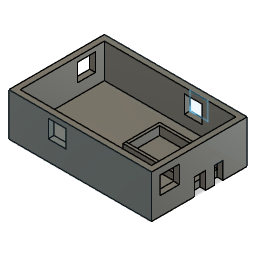
PDT LED Original Bottom Array Case v4 (Autodesk Fusion 360 design; units mm, degrees)
Autodesk Fusion 360 part; units mm, degrees
sketch "Sketch1" plane through (0, 0, 0) normal (0, 1, 0) x (1, 0, 0)
  line L0 (0, 0) -> (250, 0)
  line L1 (250, 0) -> (250, -150)
  line L2 (250, -150) -> (0, -150)
  line L3 (0, -150) -> (0, 0)
  constraint horizontal L0
  constraint vertical L1
  constraint horizontal L2
  constraint vertical L3
  constraint coincident L0.start L3.end
extrude "Extrude1" add sketch "Sketch1" along normal blind 75 makes body 1
move_face "OffsetFaces1" offset 17.253 1 faces at (83.3333, 25, 0) on bodies 1
shell "Shell1" thickness 10 removed faces 1 at (83.3333, 75, 38.498) on bodies 1
sketch "Sketch2" plane through (0, 10, 0) normal (0, 1, 0) x (-1, 0, 0)
  line L0 (-10, 140) -> (-240, 140)
  line L1 (-240, 140) -> (-240, -7.253)
  line L2 (-240, -7.253) -> (-10, -7.253)
  line L3 (-10, -7.253) -> (-10, 140)
  line L4 (-240, 24.5696) -> (-138.4926, 24.5696)
  line L5 (-138.4926, 24.5696) -> (-138.4926, 78.6538)
  line L6 (-138.4926, 78.6538) -> (-240, 78.6538)
  line L7 (-240, 78.6538) -> (-240, 24.5696)
  constraint horizontal L4
  constraint vertical L5
  constraint horizontal L6
  constraint vertical L7
  constraint coincident L1 L4.start
extrude "Extrude2" add sketch "Sketch2" along normal blind 25 contours L0 L1 L2 L3 L4 L5 L6 bodies 1
extrude "Extrude3" add 1 faces at (172.3284, 10, 42.5977) along direction (0, 1, 0) blind 22 on bodies 1 bodies 1
extrude "Extrude4" cut 1 faces at (172.3284, 32, 42.5977) along direction (0, -1, 0) blind 20 on bodies 1 bodies 1
extrude "Extrude5" cut 1 faces at (52.8309, 35, 70.4669) along direction (0, -1, 0) blind 20 on bodies 1 bodies 1
sketch "Sketch4" plane through (250, 0, 0) normal (1, 0, 0) x (0, 0, -1)
  line L0 (-150, 0) -> (17.253, 0)
  line L1 (17.253, 0) -> (17.253, 75)
  line L2 (17.253, 75) -> (-150, 75)
  line L3 (-150, 75) -> (-150, 0)
  line L4 (-25.2873, 0) -> (-40, 0)
  line L5 (-40, 0) -> (-40, 30)
  line L6 (-40, 30) -> (-25.2873, 30)
  line L7 (-25.2873, 30) -> (-25.2873, 0)
  constraint horizontal L4
  constraint vertical L5
  constraint horizontal L6
  constraint vertical L7
  constraint coincident L0 L4.start
extrude "Extrude6" cut sketch "Sketch4" against normal blind 10 contours L0 L4 L5 L6 L7 bodies 1
sketch "Sketch5" plane through (0, 30, 0) normal (0, -1, 0) x (1, 0, 0)
  line L0 (250, 25.2873) -> (250, 40)
  line L1 (250, 40) -> (240, 40)
  line L2 (240, 40) -> (240, 25.2873)
  line L3 (240, 25.2873) -> (250, 25.2873)
sketch "Sketch6" plane through (250, 0, 0) normal (1, 0, 0) x (0, 0, -1)
  line L0 (-25.2873, 30) -> (-25.2873, 0)
  line L1 (-25.2873, 0) -> (17.253, 0)
  line L2 (17.253, 0) -> (17.253, 75)
  line L3 (17.253, 75) -> (-150, 75)
  line L4 (-150, 75) -> (-150, 0)
  line L5 (-150, 0) -> (-40, 0)
  line L6 (-40, 0) -> (-40, 30)
  line L7 (-40, 30) -> (-25.2873, 30)
  line L8 (-75.3798, 0) -> (-55.2778, 0)
  line L9 (-55.2778, 0) -> (-55.2778, 30)
  line L10 (-55.2778, 30) -> (-75.3798, 30)
  line L11 (-75.3798, 30) -> (-75.3798, 0)
  constraint horizontal L8
  constraint vertical L9
  constraint horizontal L10
  constraint vertical L11
  constraint coincident L5 L8.start
extrude "Extrude7" cut sketch "Sketch6" against normal blind 10 contours L5 L8 L9 L10 L11 bodies 1
sketch "Sketch7" plane through (0, 15, 0) normal (0, 1, 0) x (-1, 0, 0)
  line L0 (-240, 24.5696) -> (-240, -7.253)
  line L1 (-240, -7.253) -> (-10, -7.253)
  line L2 (-10, -7.253) -> (-10, 140)
  line L3 (-10, 140) -> (-240, 140)
  line L4 (-240, 140) -> (-240, 78.6538)
  line L5 (-240, 78.6538) -> (-138.4926, 78.6538)
  line L6 (-138.4926, 78.6538) -> (-138.4926, 24.5696)
  line L7 (-138.4926, 24.5696) -> (-240, 24.5696)
  line L8 (-138.4926, 24.5696) -> (-133.5384, 24.5696)
  line L9 (-133.5384, 24.5696) -> (-133.5384, 78.6536)
  line L10 (-133.5384, 78.6536) -> (-138.4926, 78.6536)
  line L11 (-138.4926, 78.6536) -> (-138.4926, 24.5696)
  dimension "d22" = 54.084
  constraint horizontal L8
  constraint vertical L9
  constraint horizontal L10
  constraint vertical L11
  constraint coincident L6.end L7.start
  measures "d22" distance of L8.end L9.end
extrude "Extrude8" add sketch "Sketch7" along normal blind 5 contours L6 L8 L9 L10 L11 bodies 1
extrude "Extrude9" add 1 faces at (136.8412, 20, 60.6257) along direction (0, 1, 0) blind 7 on bodies 1 bodies 1
sketch "Sketch8" plane through (0, 0, 24.5696) normal (0, 0, 1) x (1, 0, 0)
  line L0 (240, 15) -> (138.4926, 15)
  line L1 (138.4926, 15) -> (138.4926, 12)
  line L2 (138.4926, 12) -> (240, 12)
  line L3 (240, 12) -> (240, 15)
  line L4 (240, 12) -> (138.4926, 12)
  line L5 (138.4926, 12) -> (138.4926, 24)
  line L6 (138.4926, 24) -> (240, 24)
  line L7 (240, 24) -> (240, 12)
  dimension "d27" = 12
  constraint horizontal L4
  constraint vertical L5
  constraint horizontal L6
  constraint vertical L7
  constraint coincident L2.end L3.start
  constraint coincident L1.end L2.start
  measures "d27" distance of L2.end L6.end
extrude "Extrude10" add sketch "Sketch8" against normal blind 5 separate body contours L0 L5 L6 L7 makes body 2
sketch "Sketch9" plane through (0, 0, 78.6538) normal (0, 0, -1) x (-1, 0, 0)
  line L0 (-138.4926, 15) -> (-240, 15)
  line L1 (-240, 15) -> (-240, 12)
  line L2 (-240, 12) -> (-138.4926, 12)
  line L3 (-138.4926, 12) -> (-138.4926, 15)
  line L4 (-240, 12) -> (-138.4926, 12)
  line L5 (-138.4926, 12) -> (-138.4926, 15)
  line L6 (-138.4926, 15) -> (-240, 15)
  line L7 (-240, 15) -> (-240, 12)
  line L8 (-138.4926, 12) -> (-240, 12)
  line L9 (-240, 12) -> (-240, 30)
  line L10 (-240, 30) -> (-138.4926, 30)
  line L11 (-138.4926, 30) -> (-138.4926, 12)
  constraint horizontal L4
  constraint vertical L5
  constraint horizontal L6
  constraint vertical L7
  constraint coincident L3 L0.start
  constraint coincident L1.end L2.start
  constraint horizontal L8
  constraint vertical L9
  constraint horizontal L10
  constraint vertical L11
  constraint coincident L2.end L3.start
extrude "Extrude11" add sketch "Sketch9" against normal blind 3 contours L0 L6 L9 L10 L11 bodies 1
extrude "Extrude12" add 1 faces at (172.3284, 20, 81.6538) along direction (0, 0, 1) blind 2 on bodies 1 bodies 1
extrude "Extrude13" add 1 faces at (138.4926, 24, 81.9872) along direction (-1, 0, 0) blind 5 on bodies 1 bodies 1
extrude "Extrude14" add 1 faces at (138.4926, 18, 22.903) along direction (-1, 0, 0) blind 5 on bodies 2 bodies 2 1
extrude "Extrude15" cut 1 faces at (170.6617, 30, 81.9872) along direction (0, -1, 0) blind 2 on bodies 2 bodies 2
extrude "Extrude16" cut 1 faces at (170.6617, 28, 81.9872) along direction (0, -1, 0) blind 1 on bodies 2 bodies 2
extrude "Extrude17" add 1 faces at (170.6617, 24, 21.2363) along direction (0, 1, 0) blind 3 on bodies 2 bodies 2
sketch "Sketch10" plane through (0, 0, 150) normal (0, 0, 1) x (1, 0, 0)
  line L0 (0, 0) -> (250, 0)
  line L1 (250, 0) -> (250, 75)
  line L2 (250, 75) -> (0, 75)
  line L3 (0, 75) -> (0, 0)
  line L4 (254.6404, 62.8729, -14.8751) -> (254.6404, 62.8729, -48.3239)
  line L5 (254.6404, 62.8729, -48.3239) -> (254.6404, 31.8729, -48.3239)
  line L6 (254.6404, 31.8729, -48.3239) -> (254.6404, 31.8729, -14.8751)
  line L7 (254.6404, 31.8729, -14.8751) -> (254.6404, 62.8729, -14.8751)
extrude "Extrude18" cut sketch "Sketch10" against normal blind 25 contours L4 L5 L6 L7 in plane through (254.6404, 0, 150) normal (1, 0, 0) bodies 2
sketch "Sketch11" plane through (0, 0, 150) normal (0, 0, 1) x (1, 0, 0)
  line L0 (0, 0) -> (250, 0)
  line L1 (250, 0) -> (250, 75)
  line L2 (250, 75) -> (0, 75)
  line L3 (0, 75) -> (0, 0)
  line L4 (100, 35) -> (68.9964, 35)
  line L5 (68.9964, 35) -> (68.9964, 66)
  line L6 (68.9964, 66) -> (100, 66)
  line L7 (100, 66) -> (100, 35)
  dimension "d48" = 31
  constraint horizontal L4
  constraint vertical L5
  constraint horizontal L6
  constraint vertical L7
  measures "d48" distance of L4.start L6.end
extrude "Extrude19" cut sketch "Sketch11" against normal blind 10 contours L4 L5 L6 L7 bodies 2
sketch "Sketch12" plane through (0, 0, -17.253) normal (0, 0, -1) x (-1, 0, 0)
  line L0 (-250, 0) -> (0, 0)
  line L1 (0, 0) -> (0, 75)
  line L2 (0, 75) -> (-250, 75)
  line L3 (-250, 75) -> (-250, 0)
  line L4 (6.0904, 66.4976, -25.6367) -> (6.0904, 66.4976, -56.6367)
  line L5 (6.0904, 66.4976, -56.6367) -> (6.0904, 35.265, -56.6367)
  line L6 (6.0904, 35.265, -56.6367) -> (6.0904, 35.265, -25.6367)
  line L7 (6.0904, 35.265, -25.6367) -> (6.0904, 66.4976, -25.6367)
extrude "Extrude20" cut sketch "Sketch12" against normal blind 25 contours L4 L5 L6 L7 in plane through (-6.0904, 0, -17.253) normal (-1, 0, 0) bodies 2
sketch "Sketch13" plane through (0, 0, -17.253) normal (0, 0, -1) x (-1, 0, 0)
  line L0 (-250, 0) -> (0, 0)
  line L1 (0, 0) -> (0, 75)
  line L2 (0, 75) -> (-250, 75)
  line L3 (-250, 75) -> (-250, 0)
  line L4 (-150, 65) -> (-181.0678, 65)
  line L5 (-181.0678, 65) -> (-181.0678, 34)
  line L6 (-181.0678, 34) -> (-150, 34)
  line L7 (-150, 34) -> (-150, 65)
  dimension "d54" = 31
  constraint horizontal L4
  constraint vertical L5
  constraint horizontal L6
  constraint vertical L7
  measures "d54" distance of L4.start L6.end
extrude "Extrude21" cut sketch "Sketch13" against normal blind 5 contours L4 L5 L6 L7 bodies 2
extrude "Extrude22" cut 1 faces at (170.7118, 54.6667, -12.253) along direction (0, 0, 1) blind 5 on bodies 2 bodies 2
sketch "Sketch14" plane through (0, 0, 150) normal (0, 0, 1) x (1, 0, 0)
  line L0 (68.9964, 35) -> (68.9964, 66)
  line L1 (68.9964, 66) -> (100, 66)
  line L2 (100, 66) -> (100, 35)
  line L3 (100, 35) -> (68.9964, 35)
  line L4 (0, 0) -> (250, 0)
  line L5 (250, 0) -> (250, 75)
  line L6 (250, 75) -> (0, 75)
  line L7 (0, 75) -> (0, 0)
